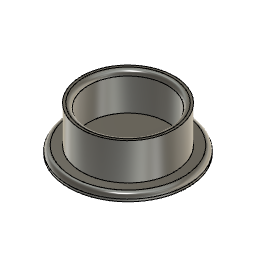
Sand timer end caps v3 (Autodesk Fusion 360 design; units mm, degrees)
Autodesk Fusion 360 part; units mm, degrees
sketch "Sketch1" plane through (0, 0, 0) normal (0, 0, 1) x (1, 0, 0)
  circle A0 centre (0, 0) radius 8.6
  circle A1 centre (0, 0) radius 10.1
  circle A2 centre (0, 0) radius 13
  dimension "d5" = 17.2
  dimension "d6" = 1.5
  dimension "d7" = 26
  constraint coincident A0.centre A1.centre
  measures "d5" diameter of A0
  measures "d7" diameter of A2
extrude "Extrude1" add sketch "Sketch1" along normal blind 8 contours A1
extrude "Extrude2" add sketch "Sketch1" against normal blind 1.5 contours A0 | A1 | A2
fillet "Fillet1" radius 1 2 edges at (-8.018, 3.1099, 8) (-12.1203, -4.701, 0)
sketch "Sketch2" plane through (0, 0, -1.5) normal (0, 0, -1) x (1, 0, 0)
  circle A0 centre (0, 0) radius 13
  line L0 (-8.9118, -8.2596) -> (7.5433, -8.2537) construction
  line L1 (7.5433, -8.2537) -> (7.5374, 8.1549) construction
  line L2 (7.5374, 8.1549) -> (-8.9176, 8.1491) construction
  line L3 (-8.9176, 8.1491) -> (-8.9118, -8.2596) construction
  dimension "d14" = 15.6
  text T0 "4" font "Arial Black" height 15.6 bold align centre middle in box 16.4551 x 16.4087 at (-8.9118, -8.2596) x (1, 0.000356) y (-0.000356, 1) spacing 1
extrude "Extrude3" cut sketch "Sketch2" against normal blind 0.5 draft -30 text T0
equation "tube_diameter = 17.2 mm"
equation "tube_height = 70 mm"
equation "base_height = 8 mm"
equation "base_diameter = 26 mm"
equation "d5 = tube_diameter"
equation "d7 = base_diameter"
equation "d8 = base_height"
equation "d14 = base_diameter * 0.6"
equation "base_label = 4"
